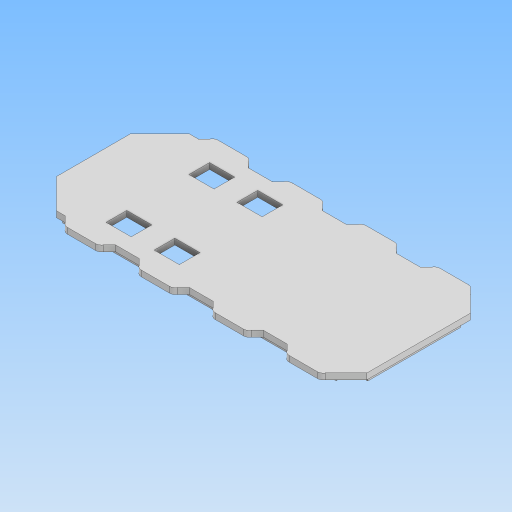
# Autodesk Inventor part: RC5 Controller kryt
Saved by Autodesk Inventor 2024 (Build 280153000, 153)
## iProperties
Created: 2024-03-14
Part Number: RC5 Controller kryt
Material: Generic
Document SubType Name: Modeling
Designer: MenMe
Density: 1 g/cm^3
Appearance: Default
Author: MenMe
Autodesk Inventor part; units mm, degrees
ref_plane "YZ Plane" through (0, 0, 0) normal (1, 0, 0) x (0, 1, 0)
ref_plane "XZ Plane" through (0, 0, 0) normal (0, 1, 0) x (-1, 0, 0)
ref_plane "XY Plane" through (0, 0, 0) normal (0, 0, 1) x (1, 0, 0)
sketch "Sketch1" plane through (0, 0, 0) normal (0, 1, 0) x (-1, 0, 0)
  arc A0 (-42.1977, 20.587) -> (-43.9298, 19.587) centre (-42.1977, 18.587) ccw
  line L0 (-45.9298, 17.587) -> (-43.9298, 19.587)
  line L1 (-50.9298, 12.587) -> (-45.9298, 17.587)
  line L2 (-50.9298, -22.413) -> (-50.9298, 12.587)
  line L3 (-43.9298, -29.413) -> (-50.9298, -22.413)
  arc A1 (-43.9298, -29.413) -> (-42.1977, -30.413) centre (-42.1977, -28.413) ccw
  line L4 (-32.6618, -30.413) -> (-42.1977, -30.413)
  arc A2 (-32.6618, -30.413) -> (-30.9298, -29.413) centre (-32.6618, -28.413) ccw
  line L5 (-28.9298, -27.413) -> (-30.9298, -29.413)
  line L6 (-20.9298, -27.413) -> (-28.9298, -27.413)
  line L7 (-18.9298, -29.413) -> (-20.9298, -27.413)
  arc A3 (-18.9298, -29.413) -> (-17.1977, -30.413) centre (-17.1977, -28.413) ccw
  line L8 (-7.6618, -30.413) -> (-17.1977, -30.413)
  arc A4 (-7.6618, -30.413) -> (-5.9298, -29.413) centre (-7.6618, -28.413) ccw
  line L9 (-3.9298, -27.413) -> (-5.9298, -29.413)
  line L10 (4.0702, -27.413) -> (-3.9298, -27.413)
  line L11 (6.0702, -29.413) -> (4.0702, -27.413)
  arc A5 (6.0702, -29.413) -> (7.8023, -30.413) centre (7.8023, -28.413) ccw
  line L12 (17.3382, -30.413) -> (7.8023, -30.413)
  arc A6 (17.3382, -30.413) -> (19.0702, -29.413) centre (17.3382, -28.413) ccw
  line L13 (21.0702, -27.413) -> (19.0702, -29.413)
  line L14 (29.0702, -27.413) -> (21.0702, -27.413)
  line L15 (31.0702, -29.413) -> (29.0702, -27.413)
  arc A7 (31.0702, -29.413) -> (32.8023, -30.413) centre (32.8023, -28.413) ccw
  line L16 (42.3382, -30.413) -> (32.8023, -30.413)
  arc A8 (42.3382, -30.413) -> (44.0702, -29.413) centre (42.3382, -28.413) ccw
  line L17 (46.0702, -27.413) -> (44.0702, -29.413)
  line L18 (49.0702, -27.413) -> (46.0702, -27.413)
  line L19 (59.0702, -17.413) -> (49.0702, -27.413)
  line L20 (59.0702, 7.587) -> (59.0702, -17.413)
  line L21 (49.0702, 17.587) -> (59.0702, 7.587)
  line L22 (46.0702, 17.587) -> (49.0702, 17.587)
  line L23 (44.0702, 19.587) -> (46.0702, 17.587)
  arc A9 (44.0702, 19.587) -> (42.3382, 20.587) centre (42.3382, 18.587) ccw
  line L24 (32.8023, 20.587) -> (42.3382, 20.587)
  arc A10 (32.8023, 20.587) -> (31.0702, 19.587) centre (32.8023, 18.587) ccw
  line L25 (29.0702, 17.587) -> (31.0702, 19.587)
  line L26 (21.0702, 17.587) -> (29.0702, 17.587)
  line L27 (19.0702, 19.587) -> (21.0702, 17.587)
  arc A11 (19.0702, 19.587) -> (17.3382, 20.587) centre (17.3382, 18.587) ccw
  line L28 (7.8023, 20.587) -> (17.3382, 20.587)
  arc A12 (7.8023, 20.587) -> (6.0702, 19.587) centre (7.8023, 18.587) ccw
  line L29 (4.0702, 17.587) -> (6.0702, 19.587)
  line L30 (-3.9298, 17.587) -> (4.0702, 17.587)
  line L31 (-5.9298, 19.587) -> (-3.9298, 17.587)
  arc A13 (-5.9298, 19.587) -> (-7.6618, 20.587) centre (-7.6618, 18.587) ccw
  line L32 (-17.1977, 20.587) -> (-7.6618, 20.587)
  arc A14 (-17.1977, 20.587) -> (-18.9298, 19.587) centre (-17.1977, 18.587) ccw
  line L33 (-20.9298, 17.587) -> (-18.9298, 19.587)
  line L34 (-28.9298, 17.587) -> (-20.9298, 17.587)
  line L35 (-30.9298, 19.587) -> (-28.9298, 17.587)
  arc A15 (-30.9298, 19.587) -> (-32.6618, 20.587) centre (-32.6618, 18.587) ccw
  line L36 (-42.1977, 20.587) -> (-32.6618, 20.587)
  point P0 (0, 0)
  point P1 (59.0702, 17.587)
  constraints: 74 end point, 32 point on circle, 16 centre point
extrude "Extrusion1" add sketch "Sketch1" along normal blind 2
sketch "Sketch2" plane through (0, 2, 0) normal (0, 1, 0) x (1, 0, 0)
  line L0 (-21.0702, 27.413) -> (-29.0702, 27.413) projected
  line L1 (-28.7702, 22.413) -> (-28.7702, 15.413)
  line L2 (-21.0023, 22.413) -> (-21.0023, 15.413)
  line L3 (-28.7702, -5.587) -> (-28.7702, -12.587)
  line L4 (-21.0023, -5.587) -> (-21.0023, -12.587)
  line L5 (-37.2702, -5.587) -> (-28.7702, -5.587)
  line L6 (-21.0023, -5.587) -> (-12.5023, -5.587)
  line L7 (-12.5023, 15.413) -> (-21.0023, 15.413)
  line L8 (-28.7702, 15.413) -> (-37.2702, 15.413)
  line L9 (-37.2702, 22.413) -> (-28.7702, 22.413)
  line L10 (-21.0023, 22.413) -> (-12.5023, 22.413)
  line L11 (-12.5023, -12.587) -> (-21.0023, -12.587)
  line L12 (-28.7702, -12.587) -> (-37.2702, -12.587)
  line L13 (-37.2702, -12.587) -> (-37.2702, -5.587)
  line L14 (-37.2702, 15.413) -> (-37.2702, 22.413)
  line L15 (-12.5023, 22.413) -> (-12.5023, 15.413)
  line L16 (-12.5023, -5.587) -> (-12.5023, -12.587)
  line L17 (-29.0702, -17.587) -> (-21.0702, -17.587) projected
  line L18 (-49.0702, -17.587) -> (-46.0702, -17.587) projected
  arc A0 (42.1977, -20.587) -> (43.9298, -19.587) centre (42.1977, -18.587) ccw projected
  point P0 (0, 0)
  point P1 (-47.5702, -17.587)
  point P2 (43.1977, -20.319)
  dimension "d15" = 8.5
  dimension "d16" = 8.5
  dimension "d19" = 10.3
  dimension "d22" = 55.7
  dimension "d23" = 5
  dimension "d24" = 5
  dimension "d25" = 5
  dimension "d26" = 5
  dimension "d27" = 7
  constraints: 32 end point, 17 parallel, 8 perpendicular, 4 horizontal, 4 point on line, 1 midpoint, 1 point on circle
  measures "d15" distance of L4.start L6.end
  measures "d16" distance of L5.start L3.start
  measures "d19" distance from line of point (-47.57, -17.587) L13
  measures "d22" distance from line of point (43.198, -20.319) L16
  measures "d23" distance from line of L0.end L9
  measures "d24" distance from line of L0.start L10
  measures "d25" distance from line of L17.end L11
  measures "d26" distance from line of L17.start L12
  measures "d27" distance of L3.start L3.end
extrude "Extrusion4" cut sketch "Sketch2" against normal blind 10
sketch "Sketch4" plane through (0, 0, 0) normal (0, -1, 0) x (1, 0, 0)
  line L0 (-49.0702, 17.587) -> (-46.0702, 17.587) projected
  line L1 (28.9298, 17.587) -> (30.9298, 19.587) projected
  line L2 (-46.0702, 17.587) -> (45.9298, 17.587)
  line L3 (43.9298, 19.587) -> (50.9298, 12.587) projected
  line L4 (-44.0702, -29.413) -> (-46.0702, -27.413) projected
  line L5 (-46.0702, -27.413) -> (45.9298, -27.413)
  line L6 (50.9298, -22.413) -> (43.9298, -29.413) projected
  line L7 (-46.0702, 17.587) -> (-49.0702, 17.587)
  line L8 (-59.0702, 7.587) -> (-49.0702, 17.587) projected
  line L9 (-49.0702, 17.587) -> (-59.0702, 7.587)
  line L10 (-59.0702, -17.413) -> (-59.0702, 7.587) projected
  line L11 (-59.0702, 7.587) -> (-59.0702, -17.413)
  line L12 (-59.0702, -17.413) -> (-49.0702, -27.413)
  line L13 (-49.0702, -27.413) -> (-46.0702, -27.413)
  line L14 (45.9298, 17.587) -> (50.9298, 12.587)
  line L15 (50.9298, 12.587) -> (50.9298, -22.413) projected
  line L16 (50.9298, -22.413) -> (45.9298, -27.413)
  line L17 (50.9298, 12.587) -> (50.9298, -22.413)
  line L18 (-37.2702, -15.413) -> (-28.7702, -15.413) projected
  line L19 (-28.7702, -15.413) -> (-28.7702, -22.413) projected
  line L20 (-28.7702, -22.413) -> (-37.2702, -22.413) projected
  line L21 (-37.2702, -22.413) -> (-37.2702, -15.413) projected
  line L22 (-37.2702, 12.587) -> (-28.7702, 12.587) projected
  line L23 (-28.7702, 12.587) -> (-28.7702, 5.587) projected
  line L24 (-28.7702, 5.587) -> (-37.2702, 5.587) projected
  line L25 (-37.2702, 5.587) -> (-37.2702, 12.587) projected
  line L26 (-21.0023, -15.413) -> (-12.5023, -15.413) projected
  line L27 (-12.5023, -15.413) -> (-12.5023, -22.413) projected
  line L28 (-12.5023, -22.413) -> (-21.0023, -22.413) projected
  line L29 (-21.0023, -22.413) -> (-21.0023, -15.413) projected
  line L30 (-21.0023, 12.587) -> (-12.5023, 12.587) projected
  line L31 (-12.5023, 12.587) -> (-12.5023, 5.587) projected
  line L32 (-12.5023, 5.587) -> (-21.0023, 5.587) projected
  line L33 (-21.0023, 5.587) -> (-21.0023, 12.587) projected
  line L34 (17.1977, -30.413) -> (7.6618, -30.413) projected
  arc A0 (17.1977, -30.413) -> (18.9298, -29.413) centre (17.1977, -28.413) ccw projected
  line L35 (20.9298, -27.413) -> (18.9298, -29.413) projected
  line L36 (28.9298, -27.413) -> (20.9298, -27.413) projected
  line L37 (30.9298, -29.413) -> (28.9298, -27.413) projected
  arc A1 (30.9298, -29.413) -> (32.6618, -30.413) centre (32.6618, -28.413) ccw projected
  line L38 (42.1977, -30.413) -> (32.6618, -30.413) projected
  arc A2 (42.1977, -30.413) -> (43.9298, -29.413) centre (42.1977, -28.413) ccw projected
  line L39 (50.9298, -22.413) -> (43.9298, -29.413) projected
  line L40 (50.9298, 12.587) -> (50.9298, -22.413) projected
  line L41 (43.9298, 19.587) -> (50.9298, 12.587) projected
  arc A3 (43.9298, 19.587) -> (42.1977, 20.587) centre (42.1977, 18.587) ccw projected
  line L42 (32.6618, 20.587) -> (42.1977, 20.587) projected
  arc A4 (32.6618, 20.587) -> (30.9298, 19.587) centre (32.6618, 18.587) ccw projected
  line L43 (28.9298, 17.587) -> (30.9298, 19.587) projected
  line L44 (20.9298, 17.587) -> (28.9298, 17.587) projected
  line L45 (18.9298, 19.587) -> (20.9298, 17.587) projected
  arc A5 (18.9298, 19.587) -> (17.1977, 20.587) centre (17.1977, 18.587) ccw projected
  line L46 (7.6618, 20.587) -> (17.1977, 20.587) projected
  arc A6 (7.6618, 20.587) -> (5.9298, 19.587) centre (7.6618, 18.587) ccw projected
  line L47 (3.9298, 17.587) -> (5.9298, 19.587) projected
  line L48 (-4.0702, 17.587) -> (3.9298, 17.587) projected
  line L49 (-6.0702, 19.587) -> (-4.0702, 17.587) projected
  arc A7 (-6.0702, 19.587) -> (-7.8023, 20.587) centre (-7.8023, 18.587) ccw projected
  line L50 (-17.3382, 20.587) -> (-7.8023, 20.587) projected
  arc A8 (-17.3382, 20.587) -> (-19.0702, 19.587) centre (-17.3382, 18.587) ccw projected
  line L51 (-21.0702, 17.587) -> (-19.0702, 19.587) projected
  line L52 (-29.0702, 17.587) -> (-21.0702, 17.587) projected
  line L53 (-31.0702, 19.587) -> (-29.0702, 17.587) projected
  arc A9 (-31.0702, 19.587) -> (-32.8023, 20.587) centre (-32.8023, 18.587) ccw projected
  line L54 (-42.3382, 20.587) -> (-32.8023, 20.587) projected
  arc A10 (-42.3382, 20.587) -> (-44.0702, 19.587) centre (-42.3382, 18.587) ccw projected
  line L55 (-46.0702, 17.587) -> (-44.0702, 19.587) projected
  line L56 (-49.0702, 17.587) -> (-46.0702, 17.587) projected
  line L57 (-59.0702, 7.587) -> (-49.0702, 17.587) projected
  line L58 (-59.0702, -17.413) -> (-59.0702, 7.587) projected
  line L59 (-49.0702, -27.413) -> (-59.0702, -17.413) projected
  line L60 (-46.0702, -27.413) -> (-49.0702, -27.413) projected
  line L61 (-44.0702, -29.413) -> (-46.0702, -27.413) projected
  arc A11 (-44.0702, -29.413) -> (-42.3382, -30.413) centre (-42.3382, -28.413) ccw projected
  line L62 (-32.8023, -30.413) -> (-42.3382, -30.413) projected
  arc A12 (-32.8023, -30.413) -> (-31.0702, -29.413) centre (-32.8023, -28.413) ccw projected
  line L63 (-29.0702, -27.413) -> (-31.0702, -29.413) projected
  line L64 (-21.0702, -27.413) -> (-29.0702, -27.413) projected
  line L65 (-19.0702, -29.413) -> (-21.0702, -27.413) projected
  arc A13 (-19.0702, -29.413) -> (-17.3382, -30.413) centre (-17.3382, -28.413) ccw projected
  line L66 (-7.8023, -30.413) -> (-17.3382, -30.413) projected
  arc A14 (-7.8023, -30.413) -> (-6.0702, -29.413) centre (-7.8023, -28.413) ccw projected
  line L67 (-4.0702, -27.413) -> (-6.0702, -29.413) projected
  line L68 (3.9298, -27.413) -> (-4.0702, -27.413) projected
  line L69 (5.9298, -29.413) -> (3.9298, -27.413) projected
  arc A15 (5.9298, -29.413) -> (7.6618, -30.413) centre (7.6618, -28.413) ccw projected
  point P0 (0, 0)
  constraints: 20 end point, 6 collinear, 2 perpendicular, 2 point on line, 1 horizontal, 1 parallel
extrude "Extrusion6" add sketch "Sketch4" along normal blind 0.01 contours L0 L2 L3 L15 L6 L5 L13 L12 L10 L8
sketch "Sketch5" plane through (0, -0.01, 0) normal (0, -1, 0) x (1, 0, 0)
  line L0 (50.9298, 12.587) -> (45.9298, 17.587) projected
  line L1 (45.9298, 17.587) -> (-49.0702, 17.587) projected
  line L2 (-49.0702, 17.587) -> (-59.0702, 7.587) projected
  line L3 (-59.0702, 7.587) -> (-59.0702, -17.413) projected
  line L4 (-59.0702, -17.413) -> (-49.0702, -27.413) projected
  line L5 (-49.0702, -27.413) -> (45.9298, -27.413) projected
  line L6 (45.9298, -27.413) -> (50.9298, -22.413) projected
  line L7 (50.9298, -22.413) -> (50.9298, 12.587) projected
  line L8 (-37.2702, -15.413) -> (-28.7702, -15.413) projected
  line L9 (-28.7702, -15.413) -> (-28.7702, -22.413) projected
  line L10 (-28.7702, -22.413) -> (-37.2702, -22.413) projected
  line L11 (-37.2702, -22.413) -> (-37.2702, -15.413) projected
  line L12 (-37.2702, 12.587) -> (-28.7702, 12.587) projected
  line L13 (-28.7702, 12.587) -> (-28.7702, 5.587) projected
  line L14 (-28.7702, 5.587) -> (-37.2702, 5.587) projected
  line L15 (-37.2702, 5.587) -> (-37.2702, 12.587) projected
  line L16 (-21.0023, -15.413) -> (-12.5023, -15.413) projected
  line L17 (-12.5023, -15.413) -> (-12.5023, -22.413) projected
  line L18 (-12.5023, -22.413) -> (-21.0023, -22.413) projected
  line L19 (-21.0023, -22.413) -> (-21.0023, -15.413) projected
  line L20 (-21.0023, 12.587) -> (-12.5023, 12.587) projected
  line L21 (-12.5023, 12.587) -> (-12.5023, 5.587) projected
  line L22 (-12.5023, 5.587) -> (-21.0023, 5.587) projected
  line L23 (-21.0023, 5.587) -> (-21.0023, 12.587) projected
  line L24 (44, -24.913) -> (-48.0347, -24.913)
  line L25 (-48.0347, -24.913) -> (-56.5702, -16.3775)
  line L26 (-56.5702, -16.3775) -> (-56.5702, 6.5514)
  line L27 (-56.5702, 6.5514) -> (-48.0347, 15.087)
  line L28 (-48.0347, 15.087) -> (44, 15.087)
  line L29 (48.4298, 10.8192) -> (48.4298, -20.6453)
  line L30 (-57.5702, -16.7917) -> (-57.5702, 6.9656)
  line L31 (-57.5702, 6.9656) -> (-48.4489, 16.087)
  line L32 (-48.4489, 16.087) -> (44, 16.087)
  line L33 (49.4298, 10.8192) -> (49.4298, -20.6453)
  line L34 (44, -25.913) -> (-48.4489, -25.913)
  line L35 (-48.4489, -25.913) -> (-57.5702, -16.7917)
  line L36 (44, 15.087) -> (44, 16.087)
  line L37 (44, -24.913) -> (44, -25.913)
  line L38 (49.4298, -20.6453) -> (48.4298, -20.6453)
  line L39 (49.4298, 10.8192) -> (48.4298, 10.8192)
  point P0 (0, 0)
  dimension "d34" = 2.5
  dimension "d35" = 1.5
  constraints: 32 end point, 4 perpendicular, 3 other
  measures "d34" distance between parallel lines of L5 L24
  measures "d35" distance between parallel lines of L3 L30
extrude "Extrusion7" add sketch "Sketch5" along normal blind 2 contours L37 L34 L35 L30 L31 L32 L36 L28 L27 L26 L25 L24 | L39 L33 L38 L29
sketch "Sketch6" plane through (-57.5702, -0.01, -16.7917) normal (-1, 0, 0) x (0, 0, 1)
  line L0 (27.6109, -2) -> (-3.8536, -2) projected
  line L1 (5, 0) -> (18.7574, 0)
  line L2 (18.7574, 0) -> (18.7574, -2)
  line L3 (18.7574, -2) -> (5, -2)
  line L4 (5, -2) -> (5, 0)
  line L5 (0, 0) -> (0, -2) projected
  line L6 (23.7574, 0) -> (23.7574, -2) projected
  point P0 (16.7917, 0.01)
  point P1 (28.3431, -2)
  point P2 (-4.5858, -2)
  dimension "d38" = 5
  dimension "d39" = 5
  constraints: 8 end point, 2 parallel, 1 horizontal, 1 perpendicular, 1 point on line
  measures "d38" distance between parallel lines of L5 L4
  measures "d39" distance between parallel lines of L6 L2
extrude "Extrusion8" cut sketch "Sketch6" against normal blind 2
body "Solid1"
